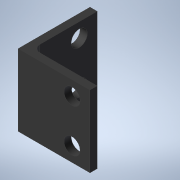
# Autodesk Inventor part: CONTROL_MONTEER
Saved by Autodesk Inventor 2020 (Build 240168000, 168)
## iProperties
Created: 2020-06-03
Part Number: CONTROL_MONTEER
Material: Generic
Document SubType Name: Modeling
Designer: Gebruiker
Density: 1 g/cm^3
Appearance: Default
Author: Gebruiker
Autodesk Inventor part; units mm, degrees
ref_plane "YZ Plane" through (0, 0, 0) normal (1, 0, 0) x (0, 1, 0)
ref_plane "XZ Plane" through (0, 0, 0) normal (0, 1, 0) x (-1, 0, 0)
ref_plane "XY Plane" through (0, 0, 0) normal (0, 0, 1) x (1, 0, 0)
sketch "Sketch1" plane through (0, 0, 0) normal (0, 0, 1) x (1, 0, 0)
  line L0 (-10, 10) -> (10, 10)
  line L1 (10, 10) -> (10, -10)
  line L2 (10, -10) -> (-10, -10)
  line L3 (-10, -10) -> (-10, 10)
  line L4 (-10, 10) -> (10, -10) construction
  line L5 (10, 10) -> (-10, -10) construction
  point P0 (0, 0)
  dimension "d0" = 20
  dimension "d1" = 20
  constraints: 12 end point, 2 midpoint, 2 parallel, 1 horizontal, 1 perpendicular
  measures "d0" distance of L1.end L2.end
  measures "d1" distance of L0.end L1.end
extrude "Extrusion1" add sketch "Sketch1" against normal blind 2
sketch "Sketch2" plane through (-10, 10, 0) normal (0, 1, 0) x (1, 0, 0)
  line L0 (20, 0) -> (0, 0) projected
  line L1 (0, 0) -> (2, 0)
  line L2 (2, 0) -> (2, 20)
  line L3 (2, 20) -> (0, 20)
  line L4 (0, 20) -> (0, 0)
  point P0 (10, 0)
  point P1 (2, 0)
  dimension "d4" = 2
  dimension "d5" = 20
  constraints: 8 end point, 2 parallel, 1 horizontal, 1 perpendicular
  measures "d4" distance of L3.end L2.end
  measures "d5" distance of L2.end L1.end
extrude "Extrusion2" add sketch "Sketch2" against normal blind 20
fillet "Fillet1" radius 2 1 edges at (-8, 0, -2)
sketch "Sketch4" plane through (0, 0, -2) normal (0, 0, -1) x (-1, 0, 0)
  circle A0 centre (-5, -6) radius 2.25
  circle A1 centre (-5, 6) radius 2.25
  line L0 (-10, -10) -> (6, -10) projected
  line L1 (6, 10) -> (-10, 10) projected
  line L2 (-10, 10) -> (-10, -10) projected
  point P0 (0, 0)
  point P1 (10, -10)
  dimension "d10" = 4.5
  dimension "d11" = 4.5
  dimension "d12" = 4
  dimension "d13" = 4
  dimension "d15" = 5
  dimension "d16" = 5
  dimension "d33" = 12
  constraints: 2 centre point
  measures "d10" diameter of A0
  measures "d11" diameter of A1
  measures "d12" distance from line of A0.centre L0
  measures "d13" distance from line of L1 A1.centre
  measures "d15" distance from line of L2 A1.centre
  measures "d16" distance from line of L2 A0.centre
  measures "d33" distance of A1.centre A0.centre
extrude "Extrusion3" cut sketch "Sketch4" against normal blind 2
sketch "Sketch5" plane through (-8, -10, -20) normal (1, 0, 0) x (0, 0, -1)
  circle A0 centre (-5, 4) radius 2.25
  circle A1 centre (-5, 16) radius 2.25
  line L0 (0, 0) -> (-16, 0) projected
  line L1 (-16, 20) -> (0, 20) projected
  line L2 (0, 20) -> (0, 0) projected
  point P0 (-20, 10)
  dimension "d19" = 4.5
  dimension "d20" = 4.5
  dimension "d21" = 4
  dimension "d23" = 5
  dimension "d24" = 5
  dimension "d38" = 4
  constraints: 2 centre point
  measures "d19" diameter of A0
  measures "d20" diameter of A1
  measures "d21" distance from line of A0.centre L0
  measures "d23" distance from line of L2 A1.centre
  measures "d24" distance from line of L2 A0.centre
  measures "d38" distance from line of L1 A1.centre
extrude "Extrusion4" cut sketch "Sketch5" against normal blind 2
body "Solid1"
